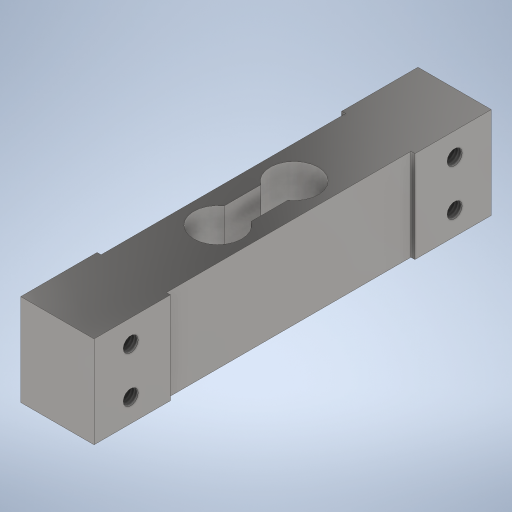
# Autodesk Inventor part: Célula de carga 2
Saved by Autodesk Inventor 2023.2 (Build 272271030, 271C)
## iProperties
Created: 2023-03-25
Part Number: Célula de carga 2
Material: Aço inoxidável
Document SubType Name: Sheet Metal
Designer: Mateus
Density: 8 g/cm^3
Sheet Metal Rule: Padrão_mm
Appearance: Aço - Polido
Mass: 518.867 g
Surface Area: 186.075 cm^2
Volume: 64.8584 cm^3
Author: Mateus
Autodesk Inventor part; units mm, degrees
ref_plane "YZ Plane" through (0, 0, 0) normal (1, 0, 0) x (0, 1, 0)
ref_plane "XZ Plane" through (0, 0, 0) normal (0, 1, 0) x (-1, 0, 0)
ref_plane "XY Plane" through (0, 0, 0) normal (0, 0, 1) x (1, 0, 0)
sketch "Esboço1" plane through (0, 0, 0) normal (0, 1, 0) x (-1, 0, 0)
  line L0 (0, 0) -> (24, 0)
  line L1 (24, -130) -> (0, -130)
  arc A0 (16.4, -59.001) -> (7.6, -59.001) centre (12, -52.5) ccw
  arc A1 (7.6, -70.999) -> (16.4, -70.999) centre (12, -77.5) ccw
  line L2 (7.6, -59.001) -> (7.6, -70.999)
  line L3 (16.4, -70.999) -> (16.4, -59.001)
  line L4 (24, -25) -> (22.7, -25)
  line L5 (22.7, -25) -> (22.7, -105)
  line L6 (22.7, -105) -> (24, -105)
  line L7 (1.3, -25.0002) -> (0, -25.0002)
  line L8 (0, -105.0002) -> (1.3, -105.0002)
  line L9 (1.3, -105.0002) -> (1.3, -25.0002)
  line L10 (24, 0) -> (24, -25)
  line L11 (24, -105) -> (24, -130)
  line L12 (0, -130) -> (0, -105.0002)
  line L13 (0, -25.0002) -> (0, 0)
  point P0 (12, 0)
  point P1 (12, -130)
  point P2 (12, -74.9986)
  point P3 (24, -65)
  point P4 (24, -65)
  point P5 (0.717, -65.0002)
  point P6 (1.3, -65.0002)
  point P7 (7.6, -65)
  dimension "d0" = 24
  dimension "d1" = 130
  dimension "d2" = 15.7
  dimension "d5" = 52.5
  dimension "d6" = 52.5
  dimension "d8" = 0
  dimension "d9" = 1.3
  dimension "d10" = 80
  dimension "d11" = 1.3
  dimension "d12" = 80
  dimension "d15" = 0
  dimension "d16" = 0
  dimension "d34" = 8.8
  dimension "d36" = 0
  dimension "d37" = 0
  dimension "d38" = 4.4
  constraints: 28 end point, 8 parallel, 4 midpoint, 4 point on circle, 3 horizontal, 3 perpendicular, 2 centre point, 2 collinear, 2 vertical, 1 equal radius
  measures "d0" distance of L1.start L1.end
  measures "d1" distance of L0.end L1.start
  measures "d2" diameter of A0
  measures "d5" distance of point (12, 0) A0.centre
  measures "d6" distance of point (12, -130) A1.centre
  measures "d8" horizontal distance of A1.centre point (12, -74.999)
  measures "d9" distance of L6.end L5.end
  measures "d10" distance of L5.end L4.end
  measures "d11" distance of L8.end L8.start
  measures "d12" distance of L8.start L7.end
  measures "d15" distance of point (24, -65) point (24, -65)
  measures "d16" vertical distance of point (0.717, -65) point (1.3, -65)
  measures "d34" distance from line of point (7.6, -65) L3
  measures "d36" horizontal distance of point (12, -130) A0.centre
  measures "d37" horizontal distance of A1.centre A0.centre
  measures "d38" horizontal distance of point (12, -74.999) point (7.6, -65)
extrude "Extrusão1" add sketch "Esboço1" along normal blind 30
sketch "Esboço2" plane through (0, 0, 0) normal (1, 0, 0) x (0, 0, -1)
  line L0 (0, 0) -> (0, 30) projected
  line L1 (130, 0) -> (130, 30) projected
  line L2 (0, 30) -> (25.0002, 30) projected
  line L3 (0, 0) -> (25.0002, 0) projected
  line L4 (105.0002, 30) -> (130, 30) projected
  line L5 (105.0002, 0) -> (130, 0) projected
  point P0 (12, 22.5)
  point P1 (12, 7.5)
  point P2 (118, 22.5)
  point P3 (118, 7.5)
  point P4 (117.5001, 0)
  dimension "d19" = 12
  dimension "d20" = 12
  dimension "d21" = 12
  dimension "d22" = 12
  dimension "d23" = 7.5
  dimension "d24" = 7.5
  dimension "d25" = 7.5
  dimension "d26" = 7.5
  constraints: 1 midpoint
  measures "d19" distance from line of L0 point (12, 22.5)
  measures "d20" distance from line of L0 point (12, 7.5)
  measures "d21" distance from line of L1 point (118, 22.5)
  measures "d22" distance from line of L1 point (118, 7.5)
  measures "d23" distance from line of L2 point (12, 22.5)
  measures "d24" distance from line of L3 point (12, 7.5)
  measures "d25" distance from line of L4 point (118, 22.5)
  measures "d26" vertical distance of point (117.5, 0) point (118, 7.5)
hole "Furo1" at (0, 22.5, -12) at (0, 7.5, -12) at (0, 22.5, -118) at (0, 7.5, -118) direction (-1, 0, 0) diameter 4.917 depth 24 tip angle 118 thread size "M6x1" class "6H" standard "ISO Metric profile"
equation "\"d38\" = 0.5 * d34"
equation "\"d20\" = d19"
equation "\"d21\" = d19"
equation "\"d22\" = d19"
equation "\"d24\" = d23"
equation "\"d25\" = d23"
equation "\"d26\" = d24"
equation "\"Raio_vergadura\" = Espessura"
equation "\"Largura_alívio_de_vergadura\" = Espessura"
equation "\"Profundidade_alívio_de_vergadura\" = 0.5 * Espessura"
equation "\"Tamanho_alívio_de_dobra\" = 4 * Espessura"
equation "\"Remanescente_mínimo\" = 2 * Espessura"
equation "\"Raiodetransição\" = Raio_vergadura"
equation "\"Tamanho_de_raio_de_Jacobi\" = Raio_vergadura"
equation "\"TamanhoFolga\" = Espessura"
equation "\"d3\" = 0.5 * d0"
equation "\"d4\" = 0.5 * d0"
equation "\"Espessura\" = 0.5"
